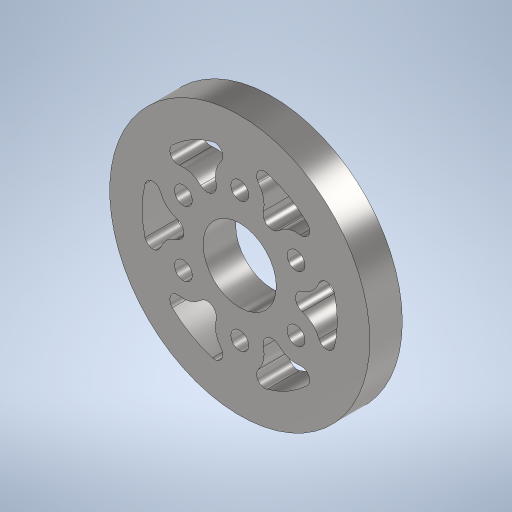
# Autodesk Inventor part: Flywheel
Saved by Autodesk Inventor 2023.2 (Build 272271000, 271)
## iProperties
Created: 2023-01-08
Part Number: Flywheel
Material: Steel, Alloy
Document SubType Name: Modeling
Designer: Nathan Cai
Density: 7.73 g/cm^3
Appearance: Semi-Polished
Mass: 71.8094 g
Surface Area: 58.2955 cm^2
Volume: 9.2897 cm^3
Author: Nathan Cai
Autodesk Inventor part; units mm, degrees
ref_plane "YZ Plane" through (0, 0, 0) normal (1, 0, 0) x (0, 1, 0)
ref_plane "XZ Plane" through (0, 0, 0) normal (0, 1, 0) x (-1, 0, 0)
ref_plane "XY Plane" through (0, 0, 0) normal (0, 0, 1) x (1, 0, 0)
sketch "Sketch1" plane through (0, 0, 0) normal (0, 0, 1) x (1, 0, 0)
  circle A0 centre (0, 0) radius 7.1437
  line L0 (0, 12.7) -> (0, 0) construction
  circle A1 centre (0, 12.7) radius 1.7526
  circle A2 centre (0, 0) radius 25.4
  circle A3 centre (0, 0) radius 19.05
  circle A4 centre (0, 12.7) radius 4.7625
  circle A5 centre (0, 0) radius 12.7 construction
  line L1 (0, 0) -> (-4.678, 11.807) construction
  circle A6 centre (-6.35, 10.9985) radius 1.8115
  circle A7 centre (-10.9985, 6.35) radius 1.7526
  circle A8 centre (-10.9985, 6.35) radius 4.7625
  circle A9 centre (-10.9985, -6.35) radius 1.7526
  circle A10 centre (-10.9985, -6.35) radius 4.7625
  circle A11 centre (0, -12.7) radius 1.7526
  circle A12 centre (0, -12.7) radius 4.7625
  circle A13 centre (10.9985, -6.35) radius 1.7526
  circle A14 centre (10.9985, -6.35) radius 4.7625
  circle A15 centre (10.9985, 6.35) radius 1.7526
  circle A16 centre (10.9985, 6.35) radius 4.7625
  circle A17 centre (-12.7, 0) radius 1.8115
  circle A18 centre (-6.35, -10.9985) radius 1.8115
  circle A19 centre (6.35, -10.9985) radius 1.8115
  circle A20 centre (12.7, 0) radius 1.8115
  circle A21 centre (6.35, 10.9985) radius 1.8115
  line L2 (2.3813, 18.9006) -> (2.3812, 16.8244)
  line L3 (-2.3812, 18.9006) -> (-2.3813, 16.8244)
  line L4 (-15.1778, 11.5125) -> (-13.3798, 10.4744)
  line L5 (-17.559, 7.3881) -> (-15.761, 6.35)
  line L6 (-17.559, -7.3881) -> (-15.761, -6.35)
  line L7 (-15.1778, -11.5125) -> (-13.3798, -10.4744)
  line L8 (-2.3813, -18.9006) -> (-2.3813, -16.8244)
  line L9 (2.3812, -18.9006) -> (2.3812, -16.8244)
  line L10 (15.1778, -11.5125) -> (13.3798, -10.4744)
  line L11 (17.559, -7.3881) -> (15.761, -6.35)
  line L12 (17.559, 7.3881) -> (15.761, 6.35)
  line L13 (15.1778, 11.5125) -> (13.3798, 10.4744)
  point P0 (-12.5642, 1.8522)
  point P1 (-7.8862, -9.9548)
  point P2 (4.678, -11.807)
  point P3 (12.5642, -1.8522)
  point P4 (7.8862, 9.9548)
  point P5 (-4.6002, 11.4674)
  point P6 (-7.6309, 9.7176)
  point P7 (15.1778, 11.5125)
  point P8 (7.6309, 9.7176)
  point P9 (4.6002, 11.4674)
  point P10 (12.2311, 1.7498)
  point P11 (15.761, 6.35)
  point P12 (17.559, 7.3881)
  point P13 (17.559, -7.3881)
  point P14 (15.761, -6.35)
  point P15 (12.2311, -1.7498)
  point P16 (7.6309, -9.7176)
  point P17 (15.1778, -11.5125)
  point P18 (2.3812, -18.9006)
  point P19 (4.6002, -11.4674)
  point P20 (-4.6002, -11.4674)
  point P21 (-2.3813, -18.9006)
  point P22 (-15.1778, -11.5125)
  point P23 (-7.6309, -9.7176)
  point P24 (-12.2311, -1.7498)
  point P25 (-17.559, -7.3881)
  point P26 (-12.2311, 1.7498)
  dimension "d0" = 14.2875
  dimension "d3" = 3.5052
  dimension "d12" = 6.35
  dimension "d13" = 50.8
  dimension "d14" = 9.525
  dimension "d19" = 25.4
  dimension "d26" = 360
  dimension "d30" = 360
  dimension "d32" = 4.7625
  dimension "d35" = 360
  constraints: 28 end point, 17 centre point, 11 coincident, 8 point on circle, 2 vertical, 1 concentric, 1 parallel, 1 tangent, 98 other
  measures "d0" diameter of A0
  measures "d3" diameter of A1
  measures "d12" radial gap between concentric circles of A2 A3
  measures "d13" diameter of A2
  measures "d14" diameter of A4
  measures "d19" diameter of A5
  measures "d32" distance between parallel lines of L3 L2
extrude "Extrusion1" add sketch "Sketch1" along normal blind 6.35 contours A2 | L12 A16 L13 A3 | A3 L10 A14 L11 | A16 | A14 | L2 A4 L3 A3 | A20 A14 A19 A12 A18 A10 A17 A8 A6 A4 A21 A16 | A3 L8 A12 L9 | A4 | A12 | L4 A8 L5 A3 | A3 L6 A10 L7 | A8 | A10
fillet "Fillet1" radius 1.5875 24 edges at (-2.3812, 18.9006, 3.175) (-2.3813, 16.8244, 3.175) (-15.1778, 11.5125, 3.175) (-13.3798, 10.4744, 3.175) (-15.761, 6.35, 3.175) (-17.559, 7.3881, 3.175) (-15.761, -6.35, 3.175) (-17.559, -7.3881, 3.175) (-13.3798, -10.4744, 3.175) (-15.1778, -11.5125, 3.175) (-2.3813, -16.8244, 3.175) (-2.3813, -18.9006, 3.175) (2.3812, -16.8244, 3.175) (2.3812, -18.9006, 3.175) (13.3798, -10.4744, 3.175) (15.1778, -11.5125, 3.175) (17.559, -7.3881, 3.175) (15.761, -6.35, 3.175) (15.761, 6.35, 3.175) (17.559, 7.3881, 3.175) (15.1778, 11.5125, 3.175) (13.3798, 10.4744, 3.175) (2.3812, 16.8244, 3.175) (2.3813, 18.9006, 3.175)
body "Solid1"
